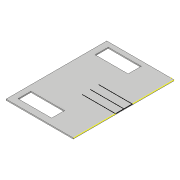
# Autodesk Inventor part: base
Saved by Autodesk Inventor 2019 (Build 230136000, 136)
## iProperties
Created: 2020-02-16
Part Number: base
Material: Generic
Document SubType Name: Modeling
Designer: Pranav naik
Density: 1 g/cm^3
Appearance: Default
Author: Pranav naik
Autodesk Inventor part; units mm, degrees
ref_plane "YZ Plane" through (0, 0, 0) normal (1, 0, 0) x (0, 1, 0)
ref_plane "XZ Plane" through (0, 0, 0) normal (0, 1, 0) x (-1, 0, 0)
ref_plane "XY Plane" through (0, 0, 0) normal (0, 0, 1) x (1, 0, 0)
sketch "Sketch1" plane through (0, 0, 0) normal (0, 0, 1) x (1, 0, 0)
  line L0 (7.6919, 0) -> (-192.3081, 0)
  line L1 (-192.3081, 0) -> (-192.3081, 3)
  line L2 (-192.3081, 3) -> (7.6919, 3)
  line L3 (7.6919, 3) -> (7.6919, 0)
  point P0 (0, 0)
  dimension "d0" = 200
  dimension "d1" = 3
  constraints: 8 end point, 2 parallel, 1 horizontal, 1 perpendicular
  measures "d0" distance of L1.end L2.end
  measures "d1" distance of L0.end L1.end
extrude "Extrusion1" add sketch "Sketch1" along normal blind 300
sketch "Sketch2" plane through (-192.3081, 3, 0) normal (0, 1, 0) x (1, 0, 0)
  line L0 (100, -149.5891) -> (200, -149.5891)
  line L1 (200, -149.5891) -> (200, -174.5891)
  line L2 (200, 0) -> (200, -300) projected
  line L3 (200, -174.5891) -> (100, -174.5891)
  line L4 (200, -149.5891) -> (200, -124.5891)
  line L5 (200, -124.5891) -> (100, -124.5891)
  point P0 (192.3081, 0)
  constraints: 10 end point, 2 horizontal, 2 point on line, 1 perpendicular
sketch "Sketch3" plane through (-192.3081, 3, 0) normal (0, 1, 0) x (1, 0, 0)
  line L0 (100.0009, -229.5915) -> (100.0009, -174.5915)
  line L1 (100.0089, -124.5986) -> (100.0089, -69.5986)
  line L2 (16.7133, -242.6689) -> (116.7133, -242.6689)
  line L3 (116.7133, -242.6689) -> (116.7133, -281.1334)
  line L4 (116.7133, -281.1334) -> (16.7133, -281.1334)
  line L5 (16.7133, -281.1334) -> (16.7133, -242.6689)
  line L6 (18.3008, -14.1302) -> (116.7133, -14.1302)
  line L7 (116.7133, -14.1302) -> (116.7133, -53.1956)
  line L8 (116.7133, -53.1956) -> (18.3008, -53.1956)
  line L9 (18.3008, -53.1956) -> (18.3008, -14.1302)
  point P0 (192.3081, 0)
  constraints: 20 end point, 4 parallel, 2 horizontal, 2 perpendicular, 2 vertical
extrude "Extrusion2" cut sketch "Sketch3" against normal blind 100
sketch "Sketch4" plane through (-192.3081, 3, 0) normal (0, 1, 0) x (1, 0, 0)
  point P0 (192.3081, 0)
body "Solid1"
